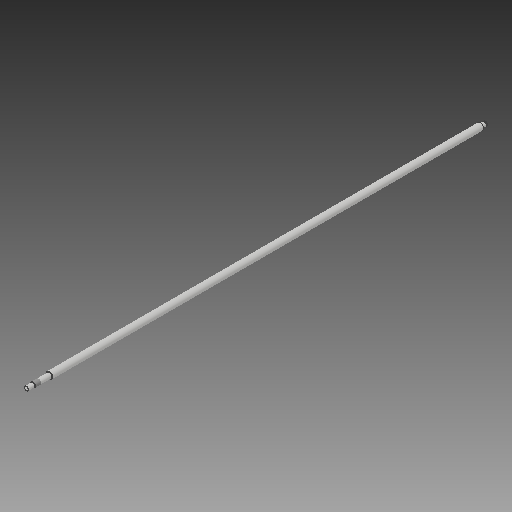
# Autodesk Inventor part: SFU16XX_Y1
Saved by Autodesk Inventor 2018 (Build 220112000, 112)
## iProperties
Created: 2018-10-24
Part Number: SFU16XX_Y1
Material: Genérico
Document SubType Name: Modeling
Designer: Georgines
Density: 1 g/cm^3
Appearance: Padrão
Author: Georgines
Autodesk Inventor part; units mm, degrees
ref_plane "YZ Plane" through (0, 0, 0) normal (1, 0, 0) x (0, 1, 0)
ref_plane "XZ Plane" through (0, 0, 0) normal (0, 1, 0) x (-1, 0, 0)
ref_plane "XY Plane" through (0, 0, 0) normal (0, 0, 1) x (1, 0, 0)
sketch "Esboço1" plane through (0, 0, 0) normal (0, 0, 1) x (1, 0, 0)
  circle A0 centre (0, 0) radius 8
  dimension "d0" = 16
  constraints: 1 centre point, 1 coincident
  measures "d0" diameter of A0
extrude "Extrusão1" add sketch "Esboço1" along normal blind 1014.5
sketch "Esboço2" plane through (0, 0, 1014.5) normal (0, 0, 1) x (1, 0, 0)
  circle A0 centre (0, 0) radius 6
  dimension "d3" = 12
  constraints: 1 centre point, 1 coincident
  measures "d3" diameter of A0
extrude "Extrusão2" add sketch "Esboço2" along normal blind 39
sketch "Esboço3" plane through (0, 0, 1053.5) normal (0, 0, 1) x (1, 0, 0)
  circle A0 centre (0, 0) radius 5
  dimension "d6" = 10
  constraints: 1 centre point, 1 coincident
  measures "d6" diameter of A0
extrude "Extrusão3" add sketch "Esboço3" along normal blind 15
sketch "Esboço4" plane through (0, 0, 0) normal (0, 0, -1) x (-1, 0, 0)
  circle A0 centre (0, 0) radius 5
  dimension "d9" = 10
  constraints: 1 centre point, 1 coincident
  measures "d9" diameter of A0
extrude "Extrusão4" add sketch "Esboço4" along normal blind 9.15
sketch "Esboço5" plane through (0, 0, -9.15) normal (0, 0, -1) x (-1, 0, 0)
  circle A0 centre (0, 0) radius 4.5
  dimension "d12" = 9
  constraints: 1 centre point, 1 coincident
  measures "d12" diameter of A0
extrude "Extrusão5" add sketch "Esboço5" along normal blind 1.15
sketch "Esboço6" plane through (0, 0, -10.3) normal (0, 0, -1) x (-1, 0, 0)
  circle A0 centre (0, 0) radius 5
  dimension "d15" = 10
  constraints: 1 centre point, 1 coincident
  measures "d15" diameter of A0
extrude "Extrusão6" add sketch "Esboço6" along normal blind 1.85
thread "Rosca1" size "M12x1.75" class "6g" standard "ANSI Metric M Profile" length 14
chamfer "Chanfro1" distance 0.5 angle 45 5 edges at (-5, 0, 1068.5) (-6, 0, 1053.5) (-8, 0, 1014.5) (-8, 0, 0) (5, 0, -12.15)
